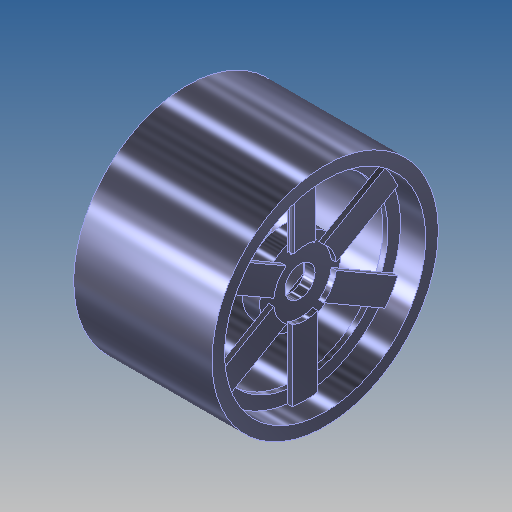
# Autodesk Inventor part: КВ33-AN1-01-02-Диск
Saved by Autodesk Inventor 2020 (Build 240168000, 168)
## iProperties
Part Number: КВ33-AN1-01-02-Диск
Material: Типовые
Document SubType Name: Modeling
Designer: sbnnl
Density: 1 g/cm^3
Appearance: Хром — полированный — синий
Mass: 83.5303 g
Surface Area: 396.977 cm^2
Volume: 83.5303 cm^3
Author: sbnnl
Autodesk Inventor part; units mm, degrees
ref_plane "YZ Plane" through (0, 0, 0) normal (1, 0, 0) x (0, 1, 0)
ref_plane "XZ Plane" through (0, 0, 0) normal (0, 1, 0) x (-1, 0, 0)
sketch "Эскиз1" plane through (0, 0, 0) normal (1, 0, 0) x (0, 1, 0)
  circle A0 centre (0, 0) radius 45
  circle A1 centre (0, 0) radius 40
  dimension "d0" = 90
  dimension "d1" = 5
  constraints: 2 centre point, 2 coincident
  measures "d0" diameter of A0
  measures "d1" radial gap between concentric circles of A0 A1
extrude "Выдавливание1" add sketch "Эскиз1" along normal blind 55
ref_plane "РабПлоскость1" through (45, 0, 0) normal (1, 0, 0) x (0, 0, -1)
sketch "Эскиз2" plane through (45, 0, 0) normal (1, 0, 0) x (0, 0, -1)
  circle A0 centre (0, 0) radius 40 projected
  circle A1 centre (0, 0) radius 35
  dimension "d5" = 5
  constraints: 1 centre point, 1 coincident
  measures "d5" radial gap between concentric circles of A0 A1
extrude "Выдавливание2" add sketch "Эскиз2" against normal blind 2
sketch "Эскиз3" plane through (45, 0, 0) normal (1, 0, 0) x (0, 0, -1)
  circle A0 centre (0, 0) radius 6
  circle A1 centre (0, 0) radius 16
  circle A2 centre (0, 0) radius 35 projected
  dimension "d19" = 12
  dimension "d20" = 32
  constraints: 2 centre point, 1 coincident, 1 concentric
  measures "d19" diameter of A0
  measures "d20" diameter of A1
extrude "Выдавливание3" add sketch "Эскиз3" against normal blind 4 contours A1
sketch "Эскиз4" plane through (45, 0, 0) normal (1, 0, 0) x (0, 0, -1)
  line L0 (-5, 42) -> (5, 42)
  line L1 (5, 42) -> (5, 11.4564)
  line L2 (-5, 11.4564) -> (-5, 42)
  line L3 (0, 0) -> (0, 36.2372) construction
  arc A0 (5, 11.4564) -> (-5, 11.4564) centre (0, 0) ccw
  dimension "d32" = 10
  dimension "d33" = 25
  dimension "d34" = 42
  constraints: 8 end point, 2 point on circle, 1 centre point, 1 coincident, 1 horizontal, 1 parallel, 1 perpendicular, 1 vertical, 1 other
  measures "d32" distance between parallel lines of L1 L2
  measures "d33" diameter of A0
  measures "d34" distance from line of L3.start L0
extrude "Выдавливание4" add sketch "Эскиз4" along normal blind 2
fillet "Сопряжение1" radius 1 5 edges at (46, 11.4564, -5) (46, 11.4564, 5) (47, 25.5714, 5) (47, 12.5, 0) (47, 25.5714, -5)
pattern_circular "Круговой массив1" count 6 over 360 about axis through (45, 0, 0) along (-1, 0, 0) of "Выдавливание4"
sketch "Эскиз5" plane through (41, 0, 0) normal (-1, 0, 0) x (0, 0, 1)
  line L0 (0, 9.815) -> (8.5, 4.9075)
  line L1 (8.5, 4.9075) -> (8.5, -4.9075)
  line L2 (8.5, -4.9075) -> (0, -9.815)
  line L3 (0, -9.815) -> (-8.5, -4.9075)
  line L4 (-8.5, -4.9075) -> (-8.5, 4.9075)
  line L5 (-8.5, 4.9075) -> (0, 9.815)
  circle A0 centre (0, 0) radius 16
  circle A1 centre (0, 0) radius 16 projected
  dimension "d41" = 17
  constraints: 12 end point, 2 coincident, 1 centre point, 1 concentric, 1 vertical, 13 other
  measures "d41" distance between parallel lines of L1 L4
extrude "Выдавливание5" add sketch "Эскиз5" along normal blind 3
